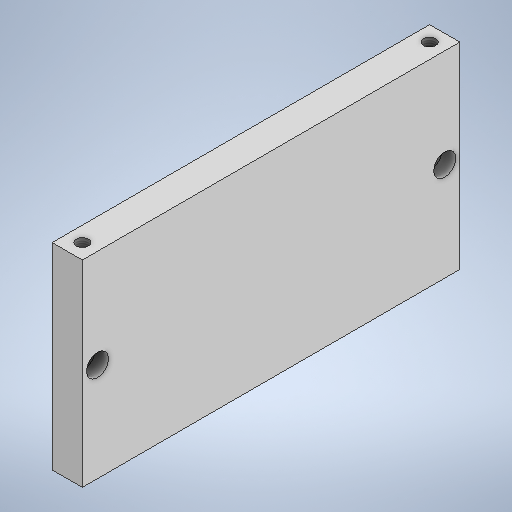
# Autodesk Inventor part: Rb PEEK - Largo
Saved by Autodesk Inventor 2025.3 (Build 293356000, 356)
## iProperties
Created: 2025-05-09
Part Number: Rb PEEK - Largo
Material: Generic
Document SubType Name: Modeling
Designer: E. Moreno
Density: 1 g/cm^3
Appearance: Default
Author: E. Moreno
Title: Rb PEEK - Largo
Autodesk Inventor part; units mm, degrees
ref_plane "YZ Plane" through (0, 0, 0) normal (1, 0, 0) x (0, 1, 0)
ref_plane "XZ Plane" through (0, 0, 0) normal (0, 1, 0) x (-1, 0, 0)
ref_plane "XY Plane" through (0, 0, 0) normal (0, 0, 1) x (1, 0, 0)
sketch "Sketch1" plane through (0, 0, 0) normal (1, 0, 0) x (0, 1, 0)
  line L0 (-32.6, 62.5) -> (32.6, 62.5)
  line L1 (32.6, 62.5) -> (32.6, -62.5)
  line L2 (32.6, -62.5) -> (-32.6, -62.5)
  line L3 (-32.6, -62.5) -> (-32.6, 62.5)
  line L4 (-32.6, 62.5) -> (32.6, -62.5) construction
  line L5 (32.6, 62.5) -> (-32.6, -62.5) construction
  point P0 (0, 0)
  dimension "d0" = 65.2
  dimension "d1" = 125
  constraints: 12 end point, 2 midpoint, 2 parallel, 1 horizontal, 1 perpendicular
  measures "d0" distance of L1.end L2.end
  measures "d1" distance of L0.end L1.end
extrude "Extrusion1" add sketch "Sketch1" along normal blind 10
sketch "Sketch2" plane through (0, 32.6, 62.5) normal (0, 1, 0) x (1, 0, 0)
  line L0 (0, 0) -> (10, 0) projected
  line L1 (0, 0) -> (5, 0)
  line L2 (5, 0) -> (5, 5)
  circle A0 centre (5, 5) radius 2
  line L3 (0, 62.5) -> (10, 62.5)
  line L4 (0, 125) -> (10, 125)
  line L5 (0, 125) -> (5, 125)
  line L6 (5, 125) -> (5, 120)
  circle A1 centre (5, 120) radius 2
  dimension "d4" = 5
  dimension "d5" = 5
  dimension "d6" = 4
  constraints: 12 end point, 5 symmetric about line, 2 centre point, 2 coincident, 1 horizontal, 1 midpoint, 1 perpendicular, 1 other
  measures "d4" distance of L0.start L1.end
  measures "d5" distance of L1.end L2.end
  measures "d6" diameter of A0
extrude "Extrusion2" cut sketch "Sketch2" against normal blind 25
thread "Thread1" size "M4x0.7" class "6H" standard "ANSI Metric M Profile" full length
thread "Thread2" size "M4x0.7" class "6H" standard "ANSI Metric M Profile" full length
sketch "Sketch3" plane through (0, -32.6, -62.5) normal (0, -1, 0) x (1, 0, 0)
  line L0 (0, 62.5) -> (9.9068, 62.5)
  line L1 (10, 0) -> (10, 125) projected
  line L2 (10, 125) -> (5, 125)
  line L3 (0, 125) -> (10, 125) projected
  line L4 (5, 125) -> (5, 120)
  circle A0 centre (5, 120) radius 2
  line L5 (10, 0) -> (5, 0)
  line L6 (0, 0) -> (10, 0)
  line L7 (5, 0) -> (5, 5)
  circle A1 centre (5, 5) radius 2
  dimension "d13" = 5
  dimension "d14" = 5
  dimension "d15" = 4
  constraints: 12 end point, 4 symmetric about line, 2 centre point, 2 coincident, 1 horizontal, 1 midpoint, 1 perpendicular, 1 other
  measures "d13" distance of L1.end L2.end
  measures "d14" distance of L2.end L4.end
  measures "d15" diameter of A0
extrude "Extrusion3" cut sketch "Sketch3" against normal blind 25
sketch "Sketch4" plane through (10, 0, 0) normal (1, 0, 0) x (0, 0, -1)
  line L0 (-62.5, 32.6) -> (-62.5, -32.6) projected
  line L1 (-62.5, 0) -> (-57.5, 0)
  circle A0 centre (-57.5, 0) radius 2
  line L2 (-62.5, -32.6) -> (62.5, -32.6) projected
  line L3 (0, -32.6) -> (0, 32.6)
  line L4 (62.5, 32.6) -> (-62.5, 32.6) projected
  line L5 (62.5, 0) -> (57.5, 0)
  circle A1 centre (57.5, 0) radius 2
  point P0 (0, 0)
  dimension "d18" = 5
  dimension "d19" = 4
  constraints: 6 end point, 3 midpoint, 3 symmetric about line, 2 centre point, 2 coincident, 1 horizontal, 1 other
  measures "d18" distance of L1.start L1.end
  measures "d19" diameter of A0
extrude "Extrusion4" cut sketch "Sketch4" against normal blind 10 contours A0 | A1
sketch "Sketch5" plane through (10, 0, 0) normal (1, 0, 0) x (0, 0, -1)
  circle A0 centre (-57.5, 0) radius 3.61
  circle A1 centre (-57.5, 0) radius 2 projected
  line L0 (0, 33.0095) -> (0, -32.6)
  line L1 (-62.5, -32.6) -> (62.5, -32.6) projected
  circle A2 centre (57.5, 0) radius 3.61
  circle A3 centre (57.5, 0) radius 2
  point P0 (0, 0)
  dimension "d22" = 7.22
  constraints: 3 centre point, 2 end point, 2 symmetric about line, 1 concentric, 1 midpoint, 2 other
  measures "d22" diameter of A0
extrude "Extrusion5" cut sketch "Sketch5" against normal blind 4.5
thread "Thread3" size "M4x0.7" class "6H" standard "ANSI Metric M Profile" full length
thread "Thread4" size "M4x0.7" class "6H" standard "ANSI Metric M Profile" full length
body "Solid1"
